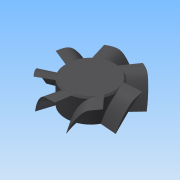
# Autodesk Inventor part: лопасти
Saved by Autodesk Inventor 2017 (Build 210142000, 142)
## iProperties
Part Number: лопасти
Material: Типовые
Document SubType Name: Modeling
Designer: alcapone
Density: 1 g/cm^3
Appearance: Серый
Mass: 1.36799 g
Surface Area: 21.7246 cm^2
Volume: 1.36799 cm^3
Author: alcapone
Autodesk Inventor part; units mm, degrees
ref_plane "XZ Plane" through (0, 0, 0) normal (0, 1, 0) x (-1, 0, 0)
ref_plane "XY Plane" through (0, 0, 0) normal (0, 0, 1) x (1, 0, 0)
sketch "Эскиз1" plane through (0, 0, 0) normal (0, 0, 1) x (1, 0, 0)
  circle A0 centre (0, 0) radius 8.5
  circle A1 centre (0, 0) radius 6.5
  circle A2 centre (0, 0) radius 1
  circle A3 centre (0, 0) radius 2
  dimension "d0" = 17
  dimension "d3" = 2
  dimension "d6" = 2
  dimension "d7" = 4
  constraints: 4 centre point, 4 coincident
  measures "d0" diameter of A0
  measures "d3" radial gap between concentric circles of A1 A0
  measures "d6" diameter of A2
  measures "d7" diameter of A3
extrude "Выдавливание1" add sketch "Эскиз1" along normal blind 8 contours A0 | A1 | A2 | A3
extrude "Выдавливание2" cut sketch "Эскиз1" along normal blind 6 contours A1 | A2 | A3
extrude "Выдавливание3" add sketch "Эскиз1" along normal blind 8 contours A3
chamfer "Фаска1" distance 0.5 angle 45 1 edges at (-8.5, 0, 8)
sketch "Эскиз3" plane through (0, 0, 0) normal (1, 0, 0) x (0, 1, 0)
  line L0 (3.5, 16) -> (3.5, -9) construction
  line L1 (3.5, -9) -> (-3.5, -9)
  line L2 (0, 0) -> (0, 16.9448) construction
  line L3 (3.5, 8) -> (2, 8) construction
  line L4 (2, 8) -> (0.7727, 7.6873) construction
  line L5 (0.7727, 7.6873) -> (0, 7.193) construction
  line L6 (0, 7.193) -> (-0.3228, 7) construction
  line L7 (-0.3228, 7) -> (-1.3074, 5.9929) construction
  line L8 (-1.3074, 5.9929) -> (-2.1419, 4.7977) construction
  line L9 (-2.1419, 4.7977) -> (-2.5709, 3.6922) construction
  line L10 (-2.5709, 3.6922) -> (-3.1239, 2.2675) construction
  line L11 (-3.1239, 2.2675) -> (-3.5, -0.0497) construction
  spline S0 degree 4 poles (3.5, 8) (2, 8) (0.7727, 7.6873) (0, 7.193) (-0.3228, 7) (-1.3074, 5.9929) (-2.1419, 4.7977) (-2.5709, 3.6922) (-3.1239, 2.2675) (-3.5, -0.0497) knots 1 1 1 1 1 2 3 4 5 6 7 7 7 7 7
  line L12 (3.5, 8) -> (2.7071, 7.5039) construction
  line L13 (2.7071, 7.5039) -> (1.2979, 6.7304) construction
  line L14 (1.2979, 6.7304) -> (0.2476, 5.9056) construction
  line L15 (0.2476, 5.9056) -> (-0.6976, 5.0185) construction
  line L16 (-0.6976, 5.0185) -> (-1.6833, 3.8614) construction
  line L17 (-1.6833, 3.8614) -> (-2, 3.3325) construction
  line L18 (-2, 3.3325) -> (-2.5709, 2.3645) construction
  line L19 (-2.5709, 2.3645) -> (-3.25, 1.0892) construction
  line L20 (-3.25, 1.0892) -> (-3.5, -0.0497) construction
  spline S1 degree 4 poles (3.5, 8) (2.7071, 7.5039) (1.2979, 6.7304) (0.2476, 5.9056) (-0.6976, 5.0185) (-1.6833, 3.8614) (-2, 3.3325) (-2.5709, 2.3645) (-3.25, 1.0892) (-3.5, -0.0497) knots 0 0 0 0 0 1 2 3 4 5 6 6 6 6 6
  point P0 (2.75, 8)
  point P1 (-3.3656, 0.4831)
  point P2 (2.75, 8)
  dimension "d13" = 7
  constraints: 16 coincident, 6 end point, 2 point on line, 1 midpoint, 1 perpendicular, 1 vertical, 7 other
  measures "d13" distance of L0.end L1.end
ref_plane "РабПлоскость1" through (18, 0, 0) normal (1, 0, 0) x (0, 1, 0)
sketch "Эскиз4" plane through (18, 0, 0) normal (1, 0, 0) x (0, 1, 0)
  line L0 (3.5, -9) -> (-3.5, -9)
  line L1 (4.7433, 8) -> (2, 8) construction
  line L2 (2, 8) -> (1.026, 7.8638) construction
  line L3 (1.026, 7.8638) -> (0.3726, 7.6604) construction
  line L4 (0.3726, 7.6604) -> (-0.5951, 7) construction
  line L5 (-0.5951, 7) -> (-1.5713, 5.8369) construction
  line L6 (-1.5713, 5.8369) -> (-2.3564, 4.7422) construction
  line L7 (-2.3564, 4.7422) -> (-3, 3.8449) construction
  line L8 (-3, 3.8449) -> (-3.9969, 1.9782) construction
  line L9 (-3.9969, 1.9782) -> (-4.973, 0) construction
  spline S0 degree 4 poles (4.7433, 8) (2, 8) (1.026, 7.8638) (0.3726, 7.6604) (-0.5951, 7) (-1.5713, 5.8369) (-2.3564, 4.7422) (-3, 3.8449) (-3.9969, 1.9782) (-4.973, 0) knots 1 1 1 1 1 2 3 4 5 6 7 7 7 7 7
  line L10 (4.7433, 8) -> (2.0756, 7.4598) construction
  line L11 (2.0756, 7.4598) -> (1.026, 6.703) construction
  line L12 (1.026, 6.703) -> (-0.3817, 5.8369) construction
  line L13 (-0.3817, 5.8369) -> (-0.903, 5.2759) construction
  line L14 (-0.903, 5.2759) -> (-1.7375, 4.3779) construction
  line L15 (-1.7375, 4.3779) -> (-2.3564, 3.5965) construction
  line L16 (-2.3564, 3.5965) -> (-2.8289, 3) construction
  line L17 (-2.8289, 3) -> (-3.621, 2) construction
  line L18 (-3.621, 2) -> (-4.973, 0) construction
  spline S1 degree 4 poles (4.7433, 8) (2.0756, 7.4598) (1.026, 6.703) (-0.3817, 5.8369) (-0.903, 5.2759) (-1.7375, 4.3779) (-2.3564, 3.5965) (-2.8289, 3) (-3.621, 2) (-4.973, 0) knots 0 0 0 0 0 1 2 3 4 5 6 6 6 6 6
  point P0 (0, 0)
  point P1 (3.3717, 8)
  point P2 (-4.2122, 1.1129)
  point P3 (3.3717, 8)
  dimension "d17" = 7
  constraints: 16 coincident, 2 end point, 1 midpoint, 7 other
  measures "d17" distance of L0.start L0.end
loft "Лофт1" add profiles "Эскиз3", "Эскиз4"
pattern_circular "Круговой массив1" count 7 over 360 about axis through (0, 0, 0) along (0, 0, 1) of "Лофт1"
sketch "Эскиз5" plane through (0, 0, 0) normal (1, 0, 0) x (0, 1, 0)
  line L0 (-20, -7) -> (19.2316, -7)
  line L1 (19.2316, -7) -> (19.2316, 0)
  line L2 (19.2316, 0) -> (-20, 0)
  line L3 (-20, 0) -> (-20, -7)
  point P0 (0, 0)
  constraints: 8 end point, 2 parallel, 1 horizontal, 1 perpendicular
extrude "Выдавливание4" cut sketch "Эскиз5" along normal mid plane 100
extrude "Выдавливание5" cut sketch "Эскиз1" along normal blind 6 contours A1
sketch "Эскиз6" plane through (0, 0, 0) normal (0, 0, 1) x (1, 0, 0)
  circle A0 centre (0, 0) radius 1 projected
  circle A1 centre (0, 0) radius 13.75
  circle A2 centre (0, 0) radius 23.031
  dimension "d29" = 27.5
  constraints: 2 centre point, 2 coincident
  measures "d29" diameter of A1
extrude "Выдавливание6" cut sketch "Эскиз6" along normal mid plane 50 contours A2
